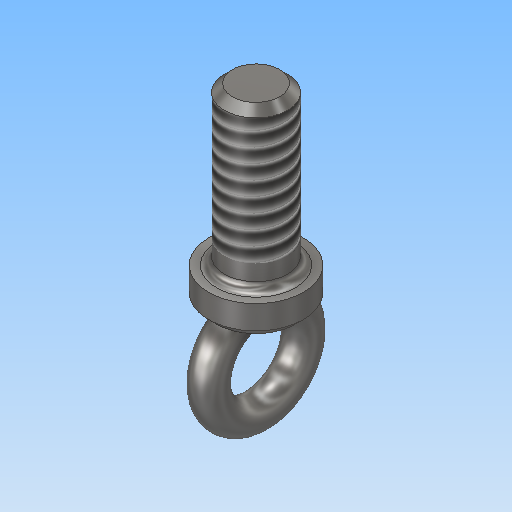
# Autodesk Inventor part: Pancake_Eye Screw
Saved by Autodesk Inventor 2018.1 (Build 221171000, 171)
## iProperties
Created: 2019-03-01
Part Number: Pancake_Eye Screw
Material: Stainless Steel
Document SubType Name: Modeling
Designer: James
Density: 8 g/cm^3
Appearance: Semi-Polished
Mass: 0.233407 g
Surface Area: 0.759261 cm^2
Volume: 0.0291759 cm^3
Author: James
Autodesk Inventor part; units mm, degrees
ref_plane "YZ Plane" through (0, 0, 0) normal (1, 0, 0) x (0, 1, 0)
ref_plane "XY Plane" through (0, 0, 0) normal (0, 0, 1) x (1, 0, 0)
sketch "Sketch1" plane through (0, 0, 0) normal (0, 0, 1) x (1, 0, 0)
  circle A0 centre (0, 1.5) radius 0.5
  line L0 (-0.7, 0) -> (0.7, 0) projected
  point P0 (0, 0)
  dimension "d0" = 1.5
  dimension "d1" = 1
  constraints: 1 centre point
  measures "d0" distance of point (0, 0) A0.centre
  measures "d1" diameter of A0
revolve "Revolution1" add sketch "Sketch1" angle 360 about axis through (-10, 0, 0) along (1, 0, 0)
ref_plane "Work Plane1" through (0, 1.5, 0) normal (0, 1, 0) x (-1, 0, 0)
sketch "Sketch2" plane through (0, 1.5, 0) normal (0, 1, 0) x (-1, 0, 0)
  circle A0 centre (0, 0) radius 1.5
  dimension "d4" = 3
  constraints: 1 centre point, 1 coincident
  measures "d4" diameter of A0
extrude "Extrusion1" add sketch "Sketch2" along normal blind 1
chamfer "Chamfer1" distance 0.25 angle 45 1 edges at (1.5, 1.5, 0)
sketch "Sketch3" plane through (0, 2.5, 0) normal (0, 1, 0) x (1, 0, 0)
  circle A0 centre (0, 0) radius 1
  dimension "d10" = 2
  constraints: 1 centre point, 1 coincident
  measures "d10" diameter of A0
extrude "Extrusion2" add sketch "Sketch3" along normal blind 5
chamfer "Chamfer2" distance 0.25 angle 45 1 edges at (-1, 7.5, 0)
thread "Thread1" size "2-56 UNC" class "2A" standard "ANSI Unified Screw Threads" length 4
fillet "Fillet1" radius 0.25 1 edges at (-1, 2.5, 0)
body "Solid1"
